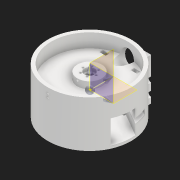
# Autodesk Inventor part: AA035b
Saved by Autodesk Inventor 2017 SP1 (Build 210196100, 196)
## iProperties
Created: 2018-03-20
Part Number: AA035b
Material: ABS Plastic
Document SubType Name: Modeling
Designer: Zach
Density: 1.06 g/cm^3
Appearance: CR White
Author: Zach
Autodesk Inventor part; units mm, degrees
sketch "Sketch1" plane through (0, 0, 0) normal (0, 0, 1) x (1, 0, 0)
  circle A0 centre (0, 0) radius 60
  circle A1 centre (0, 0) radius 5
  dimension "d0" = 120
  dimension "d1" = 10
  constraints: 2 centre point, 2 coincident
  measures "d0" diameter of A0
  measures "d1" diameter of A1
extrude "Extrusion1" add sketch "Sketch1" along normal blind 67 contours A0 | A1
sketch "Sketch2" plane through (0, 0, 0) normal (0, 1, 0) x (-1, 0, 0)
  line L0 (-60, 0) -> (60, 0) projected
  line L1 (27.5, 0) -> (-27.5, 0)
  line L2 (-27.5, 0) -> (-27.5, 61)
  line L3 (-27.5, 61) -> (27.5, 61)
  line L4 (27.5, 61) -> (27.5, 0)
  point P0 (0, 0)
  point P1 (0, 0)
  dimension "d4" = 55
  dimension "d5" = 61
  constraints: 8 end point, 2 midpoint, 2 parallel, 1 horizontal, 1 perpendicular, 1 point on line
  measures "d4" distance of L2.end L3.end
  measures "d5" distance of L1.end L2.end
extrude "Extrusion2" add sketch "Sketch2" along normal blind 61.3268
sketch "Sketch3" plane through (0, 61.3268, 0) normal (0, 1, 0) x (1, 0, 0)
  line L0 (22.5, -3.5) -> (-22.5, -3.5) construction
  line L1 (-22.5, -3.5) -> (-22.5, -43.5) construction
  line L2 (-22.5, -43.5) -> (22.5, -43.5) construction
  line L3 (22.5, -43.5) -> (22.5, -3.5) construction
  line L4 (27.5, 0) -> (-27.5, 0) construction
  circle A0 centre (-22.5, -43.5) radius 2.5
  circle A1 centre (-22.5, -3.5) radius 2.5
  circle A2 centre (22.5, -3.5) radius 2.5
  circle A3 centre (22.5, -43.5) radius 2.5
  point P0 (0, 0)
  point P1 (0, -3.5)
  point P2 (0, 0)
  dimension "d8" = 45
  dimension "d9" = 40
  dimension "d10" = 3.5
  dimension "d11" = 5
  dimension "d12" = 5
  dimension "d13" = 5
  dimension "d14" = 5
  constraints: 8 end point, 4 centre point, 4 coincident, 2 midpoint, 2 parallel, 1 horizontal, 1 perpendicular, 1 vertical alignment
  measures "d8" distance of L2.end L1.end
  measures "d9" distance of L1.end L0.end
  measures "d10" distance from line of L4 L0.end
  measures "d11" diameter of A0
  measures "d12" diameter of A1
  measures "d13" diameter of A2
  measures "d14" diameter of A3
extrude "Extrusion3" cut sketch "Sketch3" against normal blind 30
sketch "Sketch4" plane through (0, 0, 67) normal (0, 0, 1) x (1, 0, 0)
  circle A0 centre (0, 0) radius 55
  dimension "d17" = 110
  constraints: 1 centre point, 1 coincident
  measures "d17" diameter of A0
extrude "Extrusion4" cut sketch "Sketch4" against normal blind 20
sketch "Sketch5" plane through (0, 0, 47) normal (0, 0, 1) x (1, 0, 0)
  circle A0 centre (0, 0) radius 17.5
  dimension "d20" = 35
  constraints: 1 centre point, 1 coincident
  measures "d20" diameter of A0
extrude "Extrusion5" add sketch "Sketch5" along normal blind 10
sketch "Sketch6" plane through (0, 0, 57) normal (0, 0, 1) x (1, 0, 0)
  circle A0 centre (0, 0) radius 5
  dimension "d23" = 10
  constraints: 1 centre point, 1 coincident
  measures "d23" diameter of A0
extrude "Extrusion6" cut sketch "Sketch6" against normal through all
sketch "Sketch7" plane through (0, 0, 57) normal (0, 0, 1) x (1, 0, 0)
  circle A0 centre (0, 0) radius 7.5
  dimension "d26" = 15
  constraints: 1 centre point, 1 coincident
  measures "d26" diameter of A0
extrude "Extrusion7" cut sketch "Sketch7" against normal blind 5
sketch "Sketch8" plane through (0, 0, 57) normal (0, 0, 1) x (1, 0, 0)
  circle A0 centre (-9.525, 0) radius 1.5
  circle A1 centre (-4.7625, -8.2489) radius 1.5
  circle A2 centre (4.7625, -8.2489) radius 1.5
  circle A3 centre (9.525, 0) radius 1.5
  circle A4 centre (4.7625, 8.2489) radius 1.5
  circle A5 centre (-4.7625, 8.2489) radius 1.5
  point P0 (0, 0)
  dimension "d29" = 3
  dimension "d30" = 9.525
  dimension "d33" = 360
  constraints: 6 centre point, 1 horizontal alignment, 13 other
  measures "d29" diameter of A0
  measures "d30" distance of point (0, 0) A0.centre
extrude "Extrusion8" cut sketch "Sketch8" against normal blind 15
sketch "Sketch9" plane through (0, 0, 0) normal (0, 1, 0) x (-1, 0, 0)
  line L0 (-7.5, 57) -> (7.5, 57) projected
  circle A0 centre (0, 54.65) radius 1.5
  circle A1 centre (0, 59.75) radius 1.5
  line L1 (0, 59.75) -> (0, 54.65)
  line L2 (0, 58.25) -> (0, 56.15)
  point P0 (0, 0)
  point P1 (0, 57.2)
  point P2 (0, 57)
  dimension "d41" = 3
  dimension "d42" = 3
  dimension "d44" = 2.1
  dimension "d45" = 1.25
  constraints: 4 end point, 3 vertical alignment, 2 midpoint, 2 point on line, 1 vertical, 4 other
  measures "d44" distance of L2.start L2.end
  measures "d45" distance from line of L0 L2.start
extrude "Extrusion9" cut sketch "Sketch9" against normal through all
sketch "Sketch10" plane through (0, 0, 0) normal (0, 0, -1) x (-1, 0, 0)
  line L0 (0, 0) -> (-33.8074, -9.0587) construction
  line L1 (0, 0) -> (35, 0) construction
  circle A0 centre (-33.8074, -9.0587) radius 2.5
  circle A1 centre (-24.7487, 24.7487) radius 2.5
  circle A2 centre (9.0587, 33.8074) radius 2.5
  circle A3 centre (33.8074, 9.0587) radius 2.5
  circle A4 centre (24.7487, -24.7487) radius 2.5
  circle A5 centre (-9.0587, -33.8074) radius 2.5
  dimension "d48" = 35
  dimension "d49" = 165
  dimension "d50" = 5
  dimension "d53" = 360
  constraints: 6 centre point, 4 end point, 3 coincident, 1 equal length, 1 horizontal, 16 other
  measures "d48" distance of L0.start L0.end
  measures "d49" angle of L0 L1
  measures "d50" diameter of A0
extrude "Extrusion10" cut sketch "Sketch10" against normal blind 25
sketch "Sketch11" plane through (0, 0, 47) normal (0, 0, 1) x (1, 0, 0)
  line L0 (-25, 31.3268) -> (-20, 31.3268) projected
  line L1 (-25, 61.3268) -> (-20, 61.3268) projected
  line L2 (20, 31.3268) -> (25, 31.3268) projected
  line L3 (20, 61.3268) -> (25, 61.3268) projected
  line L4 (27, 41.3268) -> (18, 41.3268)
  line L5 (18, 41.3268) -> (18, 46.3268)
  line L6 (18, 46.3268) -> (27, 46.3268)
  line L7 (27, 46.3268) -> (27, 41.3268)
  line L8 (-18, 41.3268) -> (-27, 41.3268)
  line L9 (-27, 41.3268) -> (-27, 46.3268)
  line L10 (-27, 46.3268) -> (-18, 46.3268)
  line L11 (-18, 46.3268) -> (-18, 41.3268)
  point P0 (0, 0)
  point P1 (-22.5, 41.3268)
  point P2 (-22.5, 31.3268)
  point P3 (22.5, 41.3268)
  point P4 (22.5, 31.3268)
  dimension "d57" = 9
  dimension "d58" = 5
  dimension "d59" = 9
  dimension "d60" = 5
  dimension "d61" = 10
  constraints: 16 end point, 4 midpoint, 4 parallel, 2 horizontal, 2 perpendicular, 2 vertical alignment, 1 horizontal alignment
  measures "d57" distance of L5.end L6.end
  measures "d58" distance of L4.end L5.end
  measures "d59" distance of L9.end L10.end
  measures "d60" distance of L8.end L9.end
  measures "d61" distance between parallel lines of L2 L4
extrude "Extrusion11" cut sketch "Sketch11" against normal blind 8.5
sketch "Sketch12" plane through (0, 0, 0) normal (0, 0, -1) x (-1, 0, 0)
  line L0 (-27, 41.3268) -> (-18, 41.3268) projected
  line L1 (-27, 46.3268) -> (-27, 41.3268) projected
  line L2 (-18, 46.3268) -> (-27, 46.3268) projected
  line L3 (-18, 41.3268) -> (-18, 46.3268) projected
  line L4 (18, 41.3268) -> (27, 41.3268) projected
  line L5 (18, 46.3268) -> (18, 41.3268) projected
  line L6 (27, 46.3268) -> (18, 46.3268) projected
  line L7 (27, 41.3268) -> (27, 46.3268) projected
  point P0 (0, 0)
extrude "Extrusion12" cut sketch "Sketch12" against normal blind 8.5
sketch "Sketch14" plane through (0, 61.3268, 0) normal (0, 1, 0) x (1, 0, 0)
  circle A0 centre (0, -21) radius 10
  line L0 (27.5, 0) -> (-27.5, 0) projected
  point P0 (0, 0)
  point P1 (0, 0)
  dimension "d68" = 20
  dimension "d69" = 21
  constraints: 1 centre point, 1 midpoint, 1 vertical alignment
  measures "d68" diameter of A0
  measures "d69" distance of point (0, 0) A0.centre
extrude "Extrusion13" cut sketch "Sketch14" against normal blind 25
ref_plane "Work Plane2" through (19.6803, 34.0873, 0) normal (-0.866, 0.5, 0) x (0, 0, 1)
ref_plane "Work Plane1" through (-27.5, 61.3268, 0) normal (-0.866, 0.5, 0) x (0, 0, 1)
sketch "Sketch16" plane through (19.6803, 34.0873, 0) normal (-0.866, 0.5, 0) x (0, 0, 1)
  line L0 (38, -4) -> (4, -4)
  line L1 (4, -4) -> (4, -33)
  line L2 (4, -33) -> (38, -33)
  line L3 (38, -33) -> (38, -4)
  line L4 (0, 20.6394) -> (0, -99.3606) projected
  line L5 (0, 0) -> (61, 0) projected
  line L6 (17.5, -4) -> (24.5, -4)
  line L7 (24.5, -4) -> (24.5, 9)
  line L8 (24.5, 9) -> (17.5, 9)
  line L9 (17.5, 9) -> (17.5, -4)
  ellipse E0 centre (21, 13.75) end of major axis (11, 13.75) minor radius 5 construction
  point P0 (0, -39.3606)
  point P1 (0, 20.5718)
  point P2 (0, -6.9282)
  point P3 (38, -18.5)
  point P4 (21, -4)
  point P5 (21, 9)
  dimension "d74" = 34
  dimension "d75" = 29
  dimension "d81" = 33
  dimension "d82" = 7
  dimension "d83" = 13
  constraints: 16 end point, 4 midpoint, 4 parallel, 2 horizontal, 2 perpendicular, 1 point on line, 1 vertical alignment, 1 other
  measures "d74" distance of L2.end L1.end
  measures "d75" distance of L1.end L0.end
  measures "d81" distance between parallel lines of L2 L5
  measures "d82" distance of L8.end L7.end
  measures "d83" distance of L7.end L6.end
extrude "Extrusion14" cut sketch "Sketch16" along normal blind 46 and the other way blind 75 contours L3 L2 L1 L0
sketch "Sketch17" plane through (19.6803, 34.0873, 0) normal (-0.866, 0.5, 0) x (0, 0, 1)
  line L0 (38, -4) -> (5.9763, -4) projected
  line L1 (18.4882, -4) -> (25.4882, -4)
  line L2 (25.4882, -4) -> (25.4882, 9)
  line L3 (25.4882, 9) -> (18.4882, 9)
  line L4 (18.4882, 9) -> (18.4882, -4)
  point P0 (0, -39.3606)
  point P1 (5.9763, -4)
  point P2 (21.9882, -4)
  point P3 (4.5, -1)
  dimension "d84" = 7
  dimension "d85" = 13
  constraints: 8 end point, 2 parallel, 1 horizontal, 1 midpoint, 1 perpendicular, 3 other
  measures "d84" distance of L3.end L2.end
  measures "d85" distance of L2.end L1.end
extrude "Extrusion15" cut sketch "Sketch17" along normal through all both and the other way through all
sketch "Sketch18" plane through (-22.1569, 53.6232, 4) normal (-0.5, -0.866, 0) x (0.866, -0.5, 0)
  circle A0 centre (40, 26) radius 2
  circle A1 centre (7, 26) radius 2
  line L0 (7, 26) -> (40, 26) construction
  line L1 (40, 26) -> (40, 8) construction
  line L2 (40, 8) -> (7, 8) construction
  line L3 (7, 8) -> (7, 26) construction
  line L4 (0, 4.5) -> (0, 0) projected
  line L5 (0, 0) -> (0, 4.5) projected
  line L6 (0, 1.9763) -> (0, 0) projected
  line L7 (0, 34) -> (0, 21.4882) construction
  line L8 (0, 0) -> (0, 34) projected
  circle A2 centre (7, 8) radius 2
  circle A3 centre (40, 8) radius 2
  line L9 (0, 21.4882) -> (0, 14.4882) projected
  line L10 (0, 14.4882) -> (0, 1.9763) projected
  point P0 (46, -4)
  point P1 (7, 17)
  point P2 (0, 17)
  dimension "d90" = 4
  dimension "d91" = 4
  dimension "d92" = 33
  dimension "d93" = 18
  dimension "d94" = 7
  dimension "d95" = 4
  dimension "d96" = 4
  constraints: 8 end point, 4 centre point, 3 coincident, 2 midpoint, 2 parallel, 1 horizontal, 1 horizontal alignment, 1 perpendicular
  measures "d90" diameter of A0
  measures "d91" diameter of A1
  measures "d92" distance of L1.end L2.end
  measures "d93" distance of L0.end L1.end
  measures "d94" distance between parallel lines of L8 L3
  measures "d95" diameter of A2
  measures "d96" diameter of A3
extrude "Extrusion16" cut sketch "Sketch18" against normal through all
ref_plane "Work Plane3" through (-19.6569, 57.9533, 4) normal (-0.5, -0.866, 0) x (0.866, -0.5, 0)
sketch "Sketch19" plane through (-19.6569, 57.9533, 4) normal (-0.5, -0.866, 0) x (0.866, -0.5, 0)
  circle A0 centre (40, 26) radius 2 projected
  circle A1 centre (7, 26) radius 2 projected
  circle A2 centre (7, 8) radius 2 projected
  circle A3 centre (40, 8) radius 2 projected
  circle A4 centre (40, 26) radius 4
  circle A5 centre (40, 8) radius 4
  circle A6 centre (7, 8) radius 4
  circle A7 centre (7, 26) radius 4
  point P0 (46, -4)
  dimension "d100" = 8
  dimension "d101" = 8
  dimension "d102" = 8
  dimension "d103" = 8
  constraints: 4 centre point, 4 coincident
  measures "d100" diameter of A4
  measures "d101" diameter of A5
  measures "d102" diameter of A6
  measures "d103" diameter of A7
extrude "Extrusion17" cut sketch "Sketch19" against normal through all contours A0 | A1 | A2 | A3 | A4 | A5 | A6 | A7
sketch "Sketch21" plane through (-24.9495, 31.3268, 4) normal (0, 0, 1) x (1, 0, 0)
  circle A0 centre (58.7569, -40.3855) radius 2.5 construction
  circle A1 centre (15.8908, 2.4806) radius 2.5 construction
  arc A2 (79.7985, -55.6493) -> (84.6086, -24.9401) centre (24.9495, -31.3268) ccw construction
  line L0 (84.6086, -24.9401) -> (52.1713, -6.2125) construction
  arc A3 (48.7783, -4.2535) -> (52.1713, -6.2125) centre (49.6982, -6.5781) ccw construction
  line L1 (48.7783, -4.2535) -> (4.899, 21.0802) construction
  line L2 (4.899, 15) -> (4.899, 21.0802) construction
  line L3 (6.9495, 15) -> (4.899, 15) construction
  line L4 (6.9495, 10) -> (6.9495, 15) construction
  line L5 (4.899, 10) -> (6.9495, 10) construction
  line L6 (4.899, 0) -> (4.899, 10) construction
  line L7 (0, 0) -> (4.899, 0) construction
  line L8 (0, 10) -> (0, 0) construction
  line L9 (-2.0505, 10) -> (0, 10) construction
  line L10 (-2.0505, 13.9078) -> (-2.0505, 10) construction
  line L11 (-2.0505, 13.9078) -> (-11.7074, -2.8184) construction
  line L12 (79.7985, -55.6493) -> (-11.7074, -2.8184) construction
  circle A4 centre (24.9495, -31.3268) radius 55 construction
  arc A5 (75.4416, -53.1339) -> (79.1123, -21.7668) centre (24.9495, -31.3268) ccw
  arc A6 (66.7097, -48.0925) -> (66.7331, -14.6197) centre (24.9495, -31.3268) ccw
  line L13 (75.4416, -53.1339) -> (66.7097, -48.0925)
  line L14 (66.7331, -14.6197) -> (79.1123, -21.7668)
  dimension "d106" = 10
  constraints: 6 point on circle, 4 end point, 4 point on line, 2 centre point, 2 collinear, 2 concentric
  measures "d106" radial gap between concentric circles of A4 A6
extrude "Extrusion18" cut sketch "Sketch21" along normal through all
ref_plane "Work Plane4" through (-27.5, 61.3268, 61) normal (0, -0.866, 0.5) x (1, 0, 0)
sketch "Sketch24" plane through (-27.5, 61.3268, 61) normal (0, -0.866, 0.5) x (1, 0, 0)
  circle A0 centre (27.5, -15) radius 10
  line L0 (0, 0) -> (55, 0) projected
  point P0 (27.5, -83.491)
  point P1 (27.5, 0)
  dimension "d117" = 20
  dimension "d118" = 15
  constraints: 1 centre point, 1 midpoint, 1 vertical alignment
  measures "d117" diameter of A0
  measures "d118" distance from line of L0 A0.centre
extrude "Extrusion20" cut sketch "Sketch24" along normal through all both and the other way through all
sketch "Sketch25" plane through (54.1628, 9.56, 38) normal (-0.5, -0.866, 0) x (0.866, -0.5, 0)
  ellipse E0 centre (-72.7898, -17) end of major axis (-72.7898, -27) minor radius 8.6603 (-77.1421, -25.6454) -> (-77.1421, -8.3546) ccw projected
  ellipse E1 centre (-62.5418, -17) end of major axis (-74.0888, -17) minor radius 10 (-53.5337, -10.7438) -> (-72.8605, -12.5118) ccw projected
  circle A0 centre (-72.7898, -17) radius 9.5
  point P0 (-42.1263, -38)
  dimension "d121" = 19
  constraints: 1 centre point, 1 coincident, 2 other
  measures "d121" diameter of A0
extrude "Extrusion21" cut sketch "Sketch25" against normal through all contours A0 E0 | E0 A0
equation "\"d24\" = d23"
body "Solid1"
